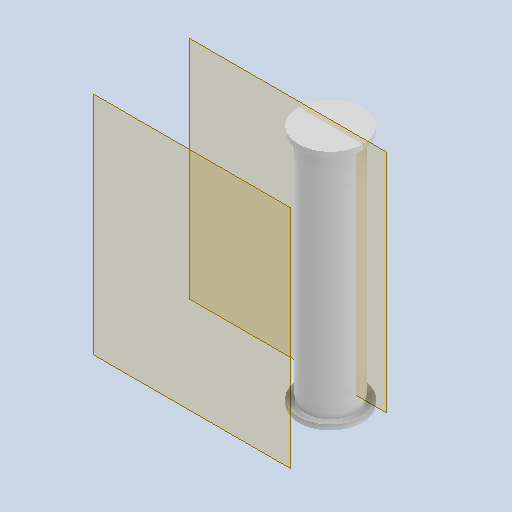
# Autodesk Inventor part: nitR3
Saved by Autodesk Inventor 2025 (Build 290162000, 162)
## iProperties
Created: 2025-02-05
Part Number: nitR3
Material: Generic
Document SubType Name: Modeling
Designer: piotr
Density: 1 g/cm^3
Appearance: Default
Author: piotr
Autodesk Inventor part; units mm, degrees
ref_plane "YZ Plane" through (0, 0, 0) normal (1, 0, 0) x (0, 1, 0)
ref_plane "XZ Plane" through (0, 0, 0) normal (0, 1, 0) x (-1, 0, 0)
ref_plane "XY Plane" through (0, 0, 0) normal (0, 0, 1) x (1, 0, 0)
ref_plane "Work Plane1" through (0, 0, 0) normal (0, 0, 1) x (1, 0, 0)
ref_plane "Work Plane2" through (0, 0, -37.5) normal (0, 0, 1) x (1, 0, 0)
sketch "Sketch1" plane through (0, 0, -37.5) normal (0, 0, 1) x (1, 0, 0)
  line L0 (41.5491, 5) -> (61.5491, 5) projected
  line L1 (41.5491, 5) -> (39.0491, 5)
  line L2 (39.0491, 5) -> (39.0491, 7)
  line L3 (39.0491, 7) -> (64.0491, 7)
  line L4 (64.0491, 7) -> (64.0491, 5)
  line L5 (64.0491, 5) -> (61.5491, 5)
  line L6 (61.5491, 5) -> (61.5491, -85)
  line L7 (61.5491, -85) -> (64.0491, -85)
  line L8 (64.0491, -85) -> (64.0491, -87)
  line L9 (64.0491, -87) -> (39.0491, -87)
  line L10 (39.0491, -87) -> (39.0491, -85)
  line L11 (39.0491, -85) -> (41.5491, -85)
  line L12 (41.5491, -85) -> (41.5491, 5)
  line L13 (51.5491, -97.5104) -> (51.5491, 34.0837)
  point P0 (0, 0)
  point P1 (51.5491, 7)
  point P2 (51.5491, -87)
  dimension "d1" = 2
  dimension "d5" = 90
  dimension "d12" = 25
  dimension "d13" = 2.5
  constraints: 26 end point, 7 point on line, 6 equal length, 3 perpendicular, 1 horizontal, 1 midpoint, 1 vertical
  measures "d1" distance of L1.end L2.end
  measures "d5" distance of L0.end L6.end
  measures "d12" distance of L2.end L3.end
  measures "d13" distance of L0.start L1.end
revolve "Revolution1" add sketch "Sketch1" angle 360 about axis through (51.5491, -97.5104, -37.5) along (0, 1, 0) contours L1 L2 L3 L13 L0 | L0 L13 L9 L10 L11 L12
body "Solid1"
